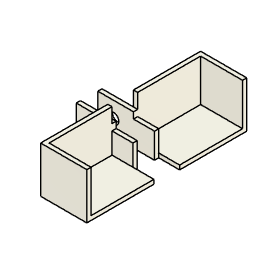
Streamdeck Plus Bracket (Autodesk Fusion 360 design; units mm, degrees)
Autodesk Fusion 360 part; units mm, degrees
sketch "front" plane through (0, 0, 0) normal (0, 0, 1) x (1, 0, 0) in component "Upper Left Bracket"
  line L0 (0, 0) -> (12, 0)
  line L1 (12, 0) -> (12, -12)
  line L2 (12, -12) -> (0, -12)
  line L3 (0, -12) -> (0, 0)
  line L4 (2, -12) -> (2, -2)
  line L5 (2, -2) -> (12, -2)
  dimension "d26" = 12
  dimension "d28" = 2
  constraint horizontal L0
  constraint vertical L1
  constraint horizontal L2
  constraint vertical L3
  constraint coincident L0.start L3.end
  constraint equal L2 L3
  constraint coincident L1 L5.end
  constraint coincident L2 L4.start
  measures "d26" distance of L0.start L2.end
sketch "back" plane through (0, 0, 0) normal (0, 0, 1) x (1, 0, 0) in component "Upper Left Bracket"
  line L0 (0, 0) -> (22, 0)
  line L1 (22, 0) -> (22, -22)
  line L2 (22, -22) -> (0, -22)
  line L3 (0, -22) -> (0, 0)
  line L4 (2, -22) -> (2, -2)
  line L5 (2, -2) -> (22, -2)
  dimension "d29" = 22
  dimension "d30" = 2
  constraint horizontal L0
  constraint vertical L1
  constraint horizontal L2
  constraint vertical L3
  constraint coincident L0.start L3.end
  constraint equal L2 L3
  constraint horizontal L5
  constraint coincident L1 L5.end
  constraint vertical L4
  constraint coincident L2 L4.start
  measures "d29" distance of L0.start L2.end
extrude "Extrude1" add sketch "back" along normal blind 30 from surface at -30 contours L0 L1 L2 L3 L4 L5 makes body 1 in component "Upper Left Bracket"
extrude "Extrude2" add sketch "back" against normal blind 2 from surface at -30 bodies 1 in component "Upper Left Bracket"
extrude "Extrude3" add sketch "front" along normal blind 2 bodies 1 in component "Upper Left Bracket"
sketch "fastener" plane through (0, 0, 0) normal (0, 0, 1) x (1, 0, 0) in component "Upper Left Bracket"
  line L0 (2, 0) -> (-15, 0)
  line L1 (-15, 0) -> (-15, -15)
  line L2 (-15, -15) -> (2, -15)
  line L3 (2, -15) -> (2, 0)
  line L4 (0, 0) -> (0, -15) construction
  circle A0 centre (-7.5, -7.5) radius 2.5
  line L5 (0, -7.5) -> (-15, -7.5) construction
  dimension "d42" = 15
  dimension "d45" = 2
  dimension "d46" = 15
  dimension "d47" = 5
  constraint horizontal L0
  constraint vertical L1
  constraint horizontal L2
  constraint vertical L3
  constraint coincident L4.start origin
  constraint coincident L2 L4.end
  constraint perpendicular L2 L4
  constraint equal L1 L4
  constraint midpoint L4 L5.start
  constraint midpoint L1 L5.end
  constraint midpoint A0.centre L5
  measures "d42" distance of L0.end L1.end
  measures "d45" distance of L3 L4
  measures "d46" distance of L1 L4
  measures "d47" diameter of A0
extrude "Extrude5" add sketch "fastener" along normal blind 2 bodies 1 in component "Upper Left Bracket"
mirror "MirrorComponent2" about plane through (0, 0, 0) normal (0, 0, 1) of bodies 1 makes body 2 in component "Upper Right Bracket"
component "Upper Left Bracket" placed x (1, 0, 0) y (0, 1, 0) z (0, 0, 1) at (0, 0, 0)
component "Upper Right Bracket" placed x (-1, 0, 0) y (0, 1, 0) z (0, 0, -1) at (0, 0, 0)
equation "d46 = d42"
